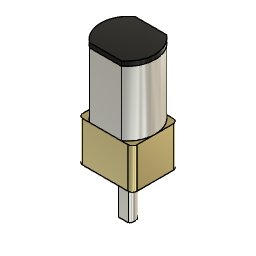
DC_Motor v3 (Autodesk Fusion 360 design; units mm, degrees)
Autodesk Fusion 360 part; units mm, degrees
sketch "Sketch1" plane through (0, 0, 0) normal (0, 0, 1) x (1, 0, 0)
  circle A0 centre (0, 0) radius 1.5
  dimension "d1" = 3
  constraint coincident A0.centre origin
  measures "d1" diameter of A0
extrude "Extrude1" add sketch "Sketch1" along normal blind 10
sketch "Sketch2" plane through (0, 0, 10) normal (0, 0, 1) x (-1, 0, 0)
  line L0 (6, -5) -> (-6, -5)
  line L1 (-6, -5) -> (-6, 5)
  line L2 (-6, 5) -> (6, 5)
  line L3 (6, 5) -> (6, -5)
  line L4 (6, -5) -> (-6, 5) construction
  line L5 (-6, -5) -> (6, 5) construction
  dimension "d4" = 10
  dimension "d5" = 12
  constraint horizontal L0
  constraint perpendicular L0 L1
  constraint parallel L0 L2
  constraint parallel L1 L3
  constraint coincident L4 origin
  constraint coincident L5 origin
  measures "d4" distance of L0.start L2.end
  measures "d5" distance of L0.start L0.end
extrude "Extrude2" add sketch "Sketch2" along normal blind 8.9
sketch "Sketch3" plane through (0, 0, 18.9) normal (0, 0, 1) x (-1, 0, 0)
  line L0 (3.5, 5) -> (-3.5, 5)
  line L1 (0, 5) -> (0, 0) construction
  line L2 (0, 0) -> (0, -5) construction
  line L3 (0, -5) -> (3.5, -5)
  line L4 (0, -5) -> (-3.5, -5)
  arc A0 (3.5, -5) -> (3.5, 5) centre (-0.25, 0) ccw
  arc A1 (-3.5, 5) -> (-3.5, -5) centre (0.25, 0) ccw
  line L5 (-6, 5) -> (-6, -5)
  line L6 (6, -5) -> (6, 5)
  point P0 (6, -5)
  point P1 (-6, -5)
  point P2 (-6, 5)
  point P3 (6, 5)
  dimension "d8" = 7
  dimension "d9" = 7
  constraint horizontal L0
  constraint midpoint L0 L1.start
  constraint coincident L1.end L2.start
  constraint perpendicular L0 L2
  constraint perpendicular L2 L3
  constraint perpendicular L2 L4
  constraint horizontal P1 L4.end
  constraint horizontal P2 L0.end
  constraint equal L3 L4
  constraint vertical L1
  constraint tangent A1 L5
  constraint tangent A0 L6
  measures "d8" distance of L0.start L0.end
  measures "d9" distance of L3.end L4.end
extrude "Extrude3" add sketch "Sketch3" along normal blind 15.3
fillet "Fillet1" radius 1 4 edges at (6, 5, 14.45) (-6, 5, 14.45) (6, -5, 14.45) (-6, -5, 14.45)
split_face "SplitFace1" 1 faces at (-1.1667, -5, 12.9667) by plane through (0, 0, 18.9) normal (0, 0, 1)
ref_plane "WorkPlane1" through (4.75, -2.5, 18.9) normal (0, 0, 1) x (1, 0, 0)
split_face "SplitFace2" 2 faces at (1.1667, -5, 12.9667) (1.1667, 5, 12.9667) by plane through (4.75, -2.5, 18.9) normal (0, 0, 1)
ref_plane "WorkPlane2" through (0, 0, 33.2) normal (0, 0, 1) x (-1, 0, 0)
split_face "SplitFace3" 4 faces at (-1.1667, -5, 24) (-6, 0, 29.1) (1.1667, 5, 24) (6, 0, 29.1) by plane through (0, 0, 33.2) normal (0, 0, 1)
sketch "Sketch4" plane through (0, 0, 0) normal (0, 0, -1) x (1, 0, 0)
  circle A0 centre (0, 0) radius 1.5
  line L0 (-1.118, 1) -> (1.118, 1)
  line L1 (0, 1.5) -> (0, 1) construction
  dimension "d16" = 0.5
  constraint coincident A0 L0.start
  constraint coincident A0 L0.end
  constraint horizontal L0
  constraint coincident A0 L1.start
  constraint midpoint L0 L1.end
  constraint vertical L1
  measures "d16" distance of L1.start L1.end
extrude "Extrude4" cut sketch "Sketch4" against normal blind 7.62 contours A0 L0 picked at (-0.3224, 1.0488)
